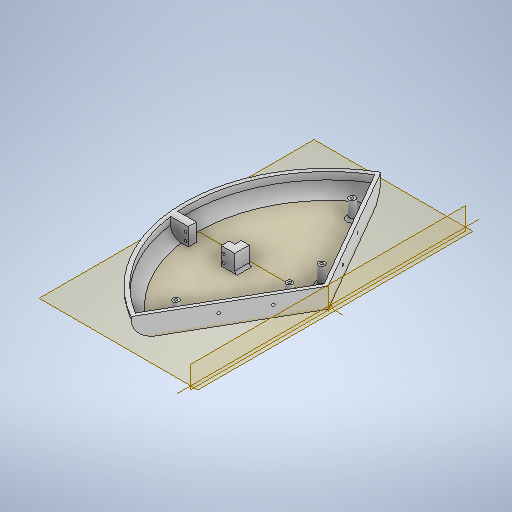
# Autodesk Inventor part: Baseplate
Saved by Autodesk Inventor 2025.1 (Build 291241000, 241)
## iProperties
Created: 2024-11-06
Part Number: Baseplate
Material: Generic
Document SubType Name: Modeling
Designer: Luke
Density: 1 g/cm^3
Appearance: Default
Author: Luke
Autodesk Inventor part; units mm, degrees
ref_plane "XY Plane" through (0, 0, 0) normal (0, 0, 1) x (1, 0, 0)
sketch "Sketch1" plane through (0, 0, 0) normal (0, 1, 0) x (-1, 0, 0)
  arc A0 (90, -155.8846) -> (90, 155.8846) centre (0, 0) ccw
  line L0 (0, 0) -> (90, 155.8846) construction
  line L1 (0, 0) -> (180, 0) construction
  line L2 (0, 0) -> (90, -155.8846) construction
  line L3 (90, -155.8846) -> (0, 0)
  line L4 (90, 155.8846) -> (0, 0)
  dimension "d3" = 180
  dimension "d4" = 60
  dimension "d5" = 120
  constraints: 10 end point, 2 point on circle, 1 centre point, 1 collinear, 1 equal length, 1 horizontal
  measures "d3" radius of A0
  measures "d4" angle of L1 L0
  measures "d5" angle of L2 L0
extrude "Extrusion1" add sketch "Sketch1" along normal blind 22
sketch "Sketch4" plane through (0, 22, 0) normal (0, 1, 0) x (1, 0, 0)
  arc A0 (-90, 155.8846) -> (-90, -155.8846) centre (0, 0) ccw projected
  line L0 (-110.5, -44) -> (-110.5, -13)
  line L1 (-110.5, -13) -> (-103.5, -13)
  line L2 (-151.5, -44) -> (-151.5, -13)
  line L3 (-151.5, -13) -> (-158.5, -13)
  line L4 (-90, -155.8846) -> (0, 0) projected
  line L5 (0, 0) -> (-90, 155.8846) projected
  line L6 (-5, 0) -> (121.9947, 0) construction
  line L7 (-5, 0) -> (45, 0) construction
  line L8 (-5, 0) -> (-85, 138.5641)
  line L9 (-5, 0) -> (155, 0) construction
  line L10 (-85, 138.5641) -> (-85, 17.3205)
  line L11 (-85, 17.3205) -> (-85, -138.5641)
  line L12 (-85, -138.5641) -> (-5, 0)
  line L13 (-110.5, -44) -> (-151.5, -44)
  line L14 (182.3936, 0) -> (-240.3989, 0) projected
  line L15 (-103.5, -13) -> (-103.5, -3)
  line L16 (-158.5, -13) -> (-158.5, -3)
  line L17 (-103.5, -3) -> (-158.5, -3)
  dimension "d43" = 160
  dimension "d98" = 13
  dimension "d99" = 55
  dimension "d101" = 41
  dimension "d102" = 110.5
  dimension "d103" = 120
  dimension "d104" = 41
  dimension "d105" = 3
  dimension "d106" = 5
  constraints: 30 end point, 4 equal length, 4 horizontal, 4 vertical, 1 collinear, 1 perpendicular, 1 other
  measures "d43" distance of L6.start L8.end
  measures "d98" distance of the line from the sketch origin of L1
  measures "d99" distance between parallel lines of L16 L15
  measures "d101" distance between parallel lines of L2 L0
  measures "d102" distance from line of L0 L4.end
  measures "d103" angle of L8 L12
  measures "d104" distance between parallel lines of L13 L17
  measures "d105" distance of the line from the sketch origin of L17
  measures "d106" distance of L6.start L4.end
extrude "Extrusion2" cut sketch "Sketch4" against normal through all contours L14 L12 L11 | L11 L10 L8 L14 | L13 L2 L3 L16 L17 L15 L1 L0
sketch "Sketch8" plane through (0, 0, 0) normal (0.8660254, 0, 0.5) x (0.5, 0, -0.8660254)
  line L0 (0, 0) -> (0, 22) projected
  line L1 (0, 11) -> (-180, 11)
  line L2 (-180, 0) -> (-180, 22) projected
  circle A0 centre (-50, 11) radius 1.65
  circle A1 centre (-100, 11) radius 1.65
  dimension "d68" = 3.3
  dimension "d69" = 3.3
  dimension "d70" = 50
  dimension "d162" = 50
  constraints: 4 midpoint, 2 centre point, 2 end point, 2 point on line
  measures "d68" diameter of A0
  measures "d69" diameter of A1
  measures "d70" distance of point (0, 11) A0.centre
  measures "d162" distance of A1.centre A0.centre
extrude "Extrusion4" cut sketch "Sketch8" against normal blind 15
sketch "Sketch9" plane through (-90, 0, -155.8846) normal (0.8660254, 0, -0.5) x (-0.5, 0, -0.8660254)
  line L0 (-180, 0) -> (-180, 11)
  line L1 (-180, 0) -> (-180, 22) projected
  line L2 (-180, 11) -> (0, 11)
  line L3 (0, 0) -> (0, 22) projected
  circle A0 centre (-130, 11) radius 1.65
  circle A1 centre (-80, 11) radius 1.65
  dimension "d74" = 3.3
  dimension "d75" = 3.3
  dimension "d76" = 50
  dimension "d161" = 50
  constraints: 4 end point, 4 midpoint, 2 centre point, 2 point on line
  measures "d74" diameter of A0
  measures "d75" diameter of A1
  measures "d76" distance of point (-180, 11) A0.centre
  measures "d161" distance of A1.centre A0.centre
extrude "Extrusion5" cut sketch "Sketch9" against normal blind 15
sketch "Sketch12" plane through (0, 0, 0) normal (0, -1, 0) x (1, 0, 0)
  arc A0 (-90, 155.8846) -> (-90, -155.8846) centre (0, 0) ccw projected
  arc A1 (-90, 155.8846) -> (-90, -155.8846) centre (0, 0) ccw
  line L0 (0, 0) -> (-90, -155.8846)
  line L1 (-90, 155.8846) -> (0, 0) projected
  line L2 (0, 0) -> (-90, 155.8846)
  constraints: 4 end point, 2 point on circle, 1 centre point, 1 coincident, 1 collinear
extrude "Extrusion8" add sketch "Sketch12" along normal blind 3
sketch "Skizze13" plane through (0, 22, 0) normal (0, 1, 0) x (1, 0, 0)
  line L0 (-75.0077, -5) -> (-158.5, -5)
  line L1 (-158.5, -5) -> (-158.5, 10)
  line L2 (-158.5, 10) -> (-75.0077, 10)
  line L3 (-75.0077, 10) -> (-75.0077, -5)
  line L4 (-158.5, -3) -> (-103.5, -3) projected
  line L5 (-158.5, -13) -> (-158.5, -3) projected
  line L6 (36, 0) -> (-216, 0) projected
  point P0 (0, 0)
  dimension "d109" = -2
  dimension "d110" = 0
  dimension "d111" = 10
  constraints: 8 end point, 2 parallel, 1 horizontal, 1 perpendicular
  measures "d109" distance between parallel lines of L4 L0
  measures "d110" distance between parallel lines of L5 L1
  measures "d111" distance between parallel lines of L2 L6
extrude "Extrusion9" cut sketch "Skizze13" against normal blind 22
sketch "Skizze15" plane through (0, 22, 0) normal (0, 1, 0) x (1, 0, 0)
  arc A0 (-91.2232, 149.343) -> (-91.2232, -149.343) centre (0, 0) ccw
  line L0 (-85, 10) -> (-85, 138.5641) projected
  line L1 (-85, 138.5641) -> (-91.2232, 149.343)
  line L2 (-85, -5) -> (-85, -138.5641) projected
  line L3 (-85, -138.5641) -> (-91.2232, -149.343)
  line L4 (-85, -5) -> (-103.5, -5) projected
  line L5 (-93.5, -5) -> (-85, -5)
  line L6 (-85, -5) -> (-85, -138.5641)
  line L7 (-93.5, -5) -> (-93.5, -23)
  line L8 (-93.5, -23) -> (-110.5, -23)
  line L9 (-110.5, -13) -> (-110.5, -44) projected
  line L10 (-151.5, -44) -> (-151.5, -13) projected
  line L11 (-110.5, -44) -> (-151.5, -44)
  line L12 (-151.5, -44) -> (-151.5, -23)
  line L13 (-151.5, -23) -> (-173.482, -23)
  line L14 (-85, 138.5641) -> (-85, 10)
  line L15 (-85, 10) -> (-158.5, 10)
  line L16 (-158.5, 10) -> (-158.5, -13)
  line L17 (-158.5, -13) -> (-174.5165, -13)
  line L18 (-158.5, 10) -> (-158.5, -13)
  line L19 (-103.5, -5) -> (-103.5, -13) projected
  line L20 (-103.5, -13) -> (-110.5, -13) projected
  line L21 (-151.5, -13) -> (-158.5, -13) projected
  dimension "d115" = 350
  dimension "d116" = 120
  dimension "d117" = 10
  dimension "d118" = 10
  dimension "d119" = 10
  constraints: 28 end point, 4 point on circle, 3 horizontal, 3 perpendicular, 3 point on line, 2 collinear, 2 vertical, 1 centre point, 1 coincident, 1 equal length
  measures "d115" diameter of A0
  measures "d116" angle of L3 L1
  measures "d117" distance between parallel lines of L7 L19
  measures "d118" distance between parallel lines of L8 L20
  measures "d119" distance between parallel lines of L13 L21
extrude "Extrusion10" cut sketch "Skizze15" against normal blind 22 contours L1 L0 L15 L16 L17 A0 | L13 L10 L11 L9 L8 L7 L4 L2 L3 A0
fillet "Rundung2" radius 13 2 edges at (-146.6555, 0, 95.4838) (-155.7023, 0, -79.8861)
fillet "Rundung3" radius 22 1 edges at (-180, -3, 0)
sketch "Skizze16" plane through (0, 0, 0) normal (0, 1, 0) x (1, 0, 0)
  circle A0 centre (-80.0555, 110) radius 4
  circle A1 centre (-28.094, 20) radius 4
  circle A2 centre (-28.094, -20) radius 4
  circle A3 centre (-80.0555, -110) radius 4
  line L0 (36, 0) -> (-216, 0) projected
  line L1 (0, 218.2384) -> (0, -218.2384) projected
  line L2 (-91.2232, 149.343) -> (-5, 0) projected
  line L3 (-5, 0) -> (-91.2232, -149.343) projected
  point P0 (0, 0)
  dimension "d127" = 10
  dimension "d128" = 8
  dimension "d129" = 8
  dimension "d130" = 10
  dimension "d131" = 90
  dimension "d132" = 20
  dimension "d133" = 8
  dimension "d134" = 8
  dimension "d135" = 90
  dimension "d136" = 20
  dimension "d137" = 10
  dimension "d138" = 10
  constraints: 4 centre point
  measures "d127" distance from line of L2 A1.centre
  measures "d128" diameter of A1
  measures "d129" diameter of A0
  measures "d130" distance from line of L2 A0.centre
  measures "d131" vertical distance of A1.centre A0.centre
  measures "d132" distance from line of L0 A1.centre
  measures "d133" diameter of A2
  measures "d134" diameter of A3
  measures "d135" vertical distance of A3.centre A2.centre
  measures "d136" distance from line of L0 A2.centre
  measures "d137" distance from line of L3 A2.centre
  measures "d138" distance from line of L3 A3.centre
extrude "Extrusion11" add sketch "Skizze16" along normal up to surface (22 mm away)
sketch "Skizze17" plane through (-80.0555, 22, -110) normal (0, 1, 0) x (1, 0, 0)
  circle A0 centre (0, 0) radius 4 projected
  circle A1 centre (0, 0) radius 1.8
  circle A2 centre (51.9615, -90) radius 4 projected
  circle A3 centre (51.9615, -90) radius 1.8
  circle A4 centre (51.9615, -130) radius 4 projected
  circle A5 centre (51.9615, -130) radius 1.8
  circle A6 centre (0, -220) radius 4 projected
  circle A7 centre (0, -220) radius 1.8
  point P0 (80.0555, -110)
  dimension "d141" = 3.6
  constraints: 4 centre point, 4 coincident, 3 equal radius
  measures "d141" diameter of A1
extrude "Extrusion12" cut sketch "Skizze17" against normal blind 5 contours A1 | A3 | A5 | A7
fillet "Rundung4" radius 3 4 edges at (-84.0555, 0, -110) (-32.094, 0, -20) (-32.094, 0, 20) (-84.0555, 0, 110)
fillet "Rundung5" radius 3 1 edges at (-93.5, 0, 14)
sketch "Skizze19" plane through (-151.5, 0, 13) normal (0, 0, -1) x (-1, 0, 0)
  circle A0 centre (-44.4, 14.8) radius 1.65
  circle A1 centre (-44.4, 4.8) radius 1.65
  circle A2 centre (3.4, 14.8) radius 1.65
  circle A3 centre (3.4, 4.8) radius 1.65
  line L0 (-41, 22) -> (-41, 0) projected
  line L1 (0, 22) -> (0, 0) projected
  line L2 (64.5, 0) -> (-187.5, 0) projected
  point P0 (-151.5, 0)
  dimension "d146" = 10
  dimension "d147" = 10
  dimension "d148" = 3.3
  dimension "d149" = 3.3
  dimension "d150" = 3.3
  dimension "d151" = 3.3
  dimension "d153" = 3.4
  dimension "d154" = 3.4
  dimension "d155" = 3.4
  dimension "d156" = 3.4
  dimension "d157" = 4.8
  dimension "d158" = 4.8
  constraints: 4 centre point
  measures "d146" distance of A3.centre A2.centre
  measures "d147" distance of A1.centre A0.centre
  measures "d148" diameter of A2
  measures "d149" diameter of A3
  measures "d150" diameter of A0
  measures "d151" diameter of A1
  measures "d153" distance from line of L0 A0.centre
  measures "d154" distance from line of L0 A1.centre
  measures "d155" distance from line of L1 A2.centre
  measures "d156" distance from line of L1 A3.centre
  measures "d157" distance from line of L2 A3.centre
  measures "d158" distance from line of L2 A1.centre
extrude "Extrusion13" cut sketch "Skizze19" against normal up to surface (10 mm away)
body "Solid1"
